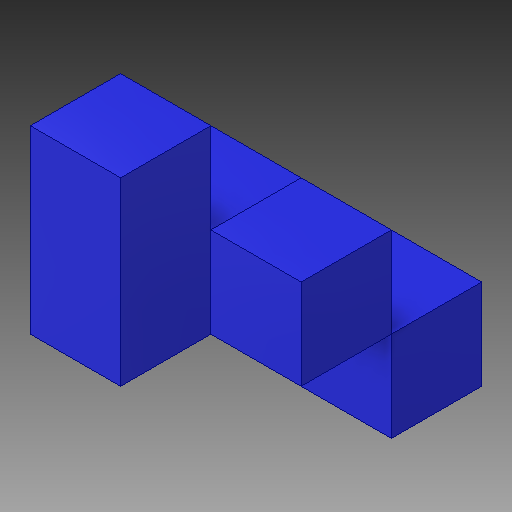
# Autodesk Inventor part: Dark Blue Part
Saved by Autodesk Inventor 2018 (Build 220112000, 112)
## iProperties
Created: 2017-11-14
Part Number: Dark Blue Part
Material: Wood (Maple)
Document SubType Name: Modeling
Designer: 232963
Density: 0.67 g/cm^3
Appearance: Blue - Wall Paint - Glossy
Mass: 27.7914 g
Surface Area: 101.613 cm^2
Volume: 41.4798 cm^3
Author: 232963
Autodesk Inventor part; units mm, degrees
ref_plane "YZ Plane" through (0, 0, 0) normal (1, 0, 0) x (0, 1, 0)
ref_plane "XZ Plane" through (0, 0, 0) normal (0, 1, 0) x (-1, 0, 0)
ref_plane "XY Plane" through (0, 0, 0) normal (0, 0, 1) x (1, 0, 0)
sketch "Sketch1" plane through (0, 0, 0) normal (0, 0, 1) x (1, 0, 0)
  line L0 (2.9023, 19.05) -> (41.0023, 19.05)
  line L1 (60.0523, 16.2003) -> (60.0523, 0)
  line L2 (60.0523, 0) -> (2.9023, 0)
  line L3 (2.9023, 0) -> (2.9023, 19.05)
  line L4 (42.0303, 0) -> (60.0523, 0)
  line L5 (60.0523, 0) -> (60.0523, 38.1)
  line L6 (60.0523, 38.1) -> (41.0023, 38.1)
  line L7 (41.0023, 38.1) -> (41.0023, 19.05)
  point P0 (0, 0)
  dimension "d0" = 57.15
  dimension "d1" = 38.1
  dimension "d2" = 19.05
  dimension "d3" = 38.1
  dimension "d4" = 19.05
  constraints: 16 end point, 4 parallel, 2 horizontal, 2 perpendicular, 2 point on line
  measures "d0" distance of L1.end L2.end
  measures "d1" distance of L4.end L5.end
  measures "d2" distance of L5.end L6.end
  measures "d3" distance of L0.start L0.end
  measures "d4" distance of L2.end L0.start
extrude "Extrusion1" add sketch "Sketch1" along normal blind 19.05
sketch "Sketch2" plane through (0, 0, 19.05) normal (0, 0, 1) x (1, 0, 0)
  line L0 (60.0523, 38.1) -> (41.0023, 38.1) projected
  line L1 (60.0523, 0) -> (60.0523, 38.1) projected
  line L2 (41.0023, 38.1) -> (60.0523, 38.1)
  line L3 (60.0523, 38.1) -> (60.0523, 19.05)
  line L4 (60.0523, 19.05) -> (41.0023, 19.05)
  line L5 (41.0023, 19.05) -> (41.0023, 38.1)
  point P0 (0, 0)
  constraints: 8 end point, 2 parallel, 1 horizontal, 1 midpoint, 1 perpendicular
extrude "Extrusion2" add sketch "Sketch2" along normal blind 19.05
sketch "Sketch3" plane through (2.9023, 0, 0) normal (-1, 0, 0) x (0, 0, 1)
  line L0 (19.05, 19.05) -> (19.05, 0) projected
  line L1 (0, 38.1) -> (38.1, 38.1) projected
  line L2 (19.05, 0) -> (38.1, 0)
  line L3 (38.1, 0) -> (38.1, 38.1)
  line L4 (38.1, 38.1) -> (19.05, 38.1)
  line L5 (19.05, 38.1) -> (19.05, 0)
  point P0 (0, 0)
  constraints: 8 end point, 2 parallel, 1 horizontal, 1 perpendicular
extrude "Extrusion3" add sketch "Sketch3" against normal blind 19.05
sketch "Sketch4" plane through (2.9023, 0, 0) normal (-1, 0, 0) x (0, 0, 1)
  line L0 (0, 0) -> (38.1, 0) projected
  line L1 (0, 19.05) -> (19.05, 19.05) projected
  line L2 (38.1, 0) -> (19.05, 0)
  line L3 (19.05, 0) -> (19.05, 19.05)
  line L4 (19.05, 19.05) -> (38.1, 19.05)
  line L5 (38.1, 19.05) -> (38.1, 0)
  constraints: 8 end point, 2 parallel, 1 horizontal, 1 perpendicular
extrude "Extrusion4" cut sketch "Sketch4" against normal blind 19.05
sketch "Sketch5" plane through (60.0523, 0, 0) normal (1, 0, 0) x (0, 0, -1)
  line L0 (-19.05, 19.05) -> (-19.05, 38.1) projected
  line L1 (0, 38.1) -> (0, 0) projected
  line L2 (-19.05, 38.1) -> (0, 38.1)
  line L3 (0, 38.1) -> (0, 19.05)
  line L4 (0, 19.05) -> (-19.05, 19.05)
  line L5 (-19.05, 19.05) -> (-19.05, 38.1)
  constraints: 8 end point, 2 parallel, 1 horizontal, 1 midpoint, 1 perpendicular
extrude "Extrusion5" cut sketch "Sketch5" against normal blind 20.6375
sketch "Sketch6" plane through (2.9023, 38.1, 19.05) normal (-1, 0, 0) x (0, 0, 1)
  line L0 (-19.05, -19.05) -> (0, -19.05) projected
  line L1 (0, -19.05) -> (19.05, -19.05)
  line L2 (19.05, -19.05) -> (19.05, -38.1)
  line L3 (19.05, -38.1) -> (0, -38.1)
  line L4 (0, -38.1) -> (0, -19.05)
  point P0 (-19.05, -38.1)
  dimension "d15" = 19.05
  dimension "d16" = 19.05
  constraints: 8 end point, 2 parallel, 1 horizontal, 1 perpendicular
  measures "d15" distance of L2.end L3.end
  measures "d16" distance of L1.end L2.end
extrude "Extrusion6" add sketch "Sketch6" against normal blind 19.05
body "Solid1"
